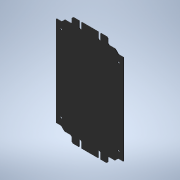
# Autodesk Inventor part: CAD_MPL_1301.000
Saved by Autodesk Inventor 2021 (Build 250183000, 183)
## iProperties
Created: 2025-05-02
Part Number: CAD_MPL_1301.000
Material: Generic
Catalog Web Link: www.cadenas.de
Description: KX EB Stainless steel Mounting plate-KX EB Stainless steel Mounting plate
Vendor: RITTAL
Document SubType Name: Modeling
Designer: psAdmin
Manufacturer: RITTAL
Mass: 92.1587 g
Surface Area: 943.235 cm^2
Volume: 92.1587 cm^3
Density: 1 g/cm^3
Appearance: PSOLRGB-175-175-175
Category: PARTsolutions
Company: RITTAL
Title: CAD_MPL_1301.000
Author: Cadenas PARTsolutions
Comments: KX EB Stainless steel Mounting plate
PSOL_IDENT_0: {$CADENAS_DATA/23d-libs/rittal/schaltschranksys/ausbauteile_cad/montageplatten/kx_eb_edel_sep_mpl.pr
PSOL_IDENT_1: j},202 {VTYP=3D},{NB=CAD_MPL_1301.000},{LINA=CAD_MPL_1301.000},{NN=KX EB Stainless steel Mounting pl
PSOL_IDENT_2: ate},{DATE=28.04.2025 21:10:25},{GEOMDATE=11.04.2025 11:21:18},{VERSION=},{LINEID=80},{WBVAR=},{WBNU
PSOL_IDENT_3: MERIC=}  {NB=CAD_MPL_1301.000},{LINA=CAD_MPL_1301.000},{KT=DUMMY},{BEST=CAD_MPL_1301.000},{BEST2=130
PSOL_IDENT_4: 1.000},{DETAIL=1},{F=175},{G=285},{S=2},{VER=4},{B1=200},{H1=300},{GEW=0}
NB: CAD_MPL_1301.000
NN: KX EB Stainless steel Mounting plate
NT: KX EB Stainless steel Mounting plate
NBSYN: $BEST.
LINA: CAD_MPL_1301.000
CATALOG: Rittal
BEST: CAD_MPL_1301.000
F: 175
G: 285
S: 2
GEW: 0
SUPPLIER: RITTAL
ARTICLENO: CAD_MPL_1301.000
BOMINFO: CAD_MPL_1301.000
CREATOR: CADENAS GmbH
Autodesk Inventor part; units mm, degrees
sketch "Sketch_7" plane through (0, 0, 0) normal (0, 0, 1) x (1, 0, 0)
  line L0 (-87.5, 117.5) -> (-87.5, -117.5)
  line L1 (-87.5, -117.5) -> (-74.5, -117.5)
  line L2 (-74.5, -117.5) -> (-66, -126)
  line L3 (-66, -126) -> (-50, -126)
  line L4 (-50, -126) -> (-47, -129)
  line L5 (-47, -129) -> (-47, -139.5)
  line L6 (-47, -139.5) -> (-44, -142.5)
  line L7 (-44, -142.5) -> (-28.3, -142.5)
  line L8 (-28.3, -142.5) -> (-28.3, -128)
  arc A0 (-21.7, -128) -> (-28.3, -128) centre (-25, -128) ccw
  line L9 (-21.7, -128) -> (-21.7, -142.5)
  line L10 (-21.7, -142.5) -> (21.7, -142.5)
  line L11 (21.7, -142.5) -> (21.7, -128)
  arc A1 (28.3, -128) -> (21.7, -128) centre (25, -128) ccw
  line L12 (28.3, -128) -> (28.3, -142.5)
  line L13 (28.3, -142.5) -> (44, -142.5)
  line L14 (44, -142.5) -> (47, -139.5)
  line L15 (47, -139.5) -> (47, -129)
  line L16 (47, -129) -> (50, -126)
  line L17 (50, -126) -> (66, -126)
  line L18 (66, -126) -> (74.5, -117.5)
  line L19 (74.5, -117.5) -> (87.5, -117.5)
  line L20 (87.5, -117.5) -> (87.5, 117.5)
  line L21 (87.5, 117.5) -> (74.5, 117.5)
  line L22 (74.5, 117.5) -> (66, 126)
  line L23 (66, 126) -> (50, 126)
  line L24 (50, 126) -> (47, 129)
  line L25 (47, 129) -> (47, 139.5)
  line L26 (47, 139.5) -> (44, 142.5)
  line L27 (44, 142.5) -> (28.3, 142.5)
  line L28 (28.3, 142.5) -> (28.3, 128)
  arc A2 (21.7, 128) -> (28.3, 128) centre (25, 128) ccw
  line L29 (21.7, 128) -> (21.7, 142.5)
  line L30 (21.7, 142.5) -> (-21.7, 142.5)
  line L31 (-21.7, 142.5) -> (-21.7, 128)
  arc A3 (-28.3, 128) -> (-21.7, 128) centre (-25, 128) ccw
  line L32 (-28.3, 128) -> (-28.3, 142.5)
  line L33 (-28.3, 142.5) -> (-44, 142.5)
  line L34 (-44, 142.5) -> (-47, 139.5)
  line L35 (-47, 139.5) -> (-47, 129)
  line L36 (-47, 129) -> (-50, 126)
  line L37 (-50, 126) -> (-66, 126)
  line L38 (-66, 126) -> (-74.5, 117.5)
  line L39 (-74.5, 117.5) -> (-87.5, 117.5)
  circle A4 centre (75, 100) radius 2.6
  circle A5 centre (75, -100) radius 2.6
  circle A6 centre (-75, 100) radius 2.6
  circle A7 centre (-75, -100) radius 2.6
  constraints: 80 end point, 8 centre point, 8 point on circle
extrude "Extrusion1" add sketch "Sketch_7" along normal blind 2
ref_plane "MONTAGEPLATTE_XY" through (0, 0, 0) normal (0, 0, 1) x (1, 0, 0)
ref_plane "MONTAGEPLATTE_YZ" through (0, 0, 0) normal (1, 0, 0) x (0, 1, 0)
ref_plane "MONTAGEPLATTE_ZX" through (0, 0, 0) normal (0, 1, 0) x (0, 0, 1)
body "Solid1"
